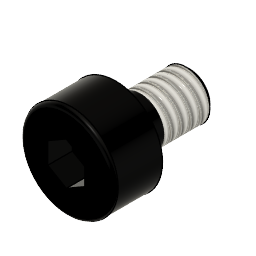
Mesh_Node (Autodesk Fusion 360 archive; units mm, degrees)
design "Hexagon Socket Head Cap Screw ISO 4762 - M2 x 3 Steel 4.6 Black"
description: Hexagon Socket Head Cap Screw ISO 4762 - M2 x 3
part number: ISO 4762 - M2 x 3 Steel 4.6 Black
Autodesk Fusion 360 part; units mm, degrees
sketch "Sketch1" plane through (0, 0, 0) normal (0, 1, 0) x (1, 0, 0)
  line L0 (-1, 0) -> (-1, 3)
  line L1 (-1, 3) -> (0, 3)
  line L2 (0, 3) -> (0, -2)
  line L3 (-1, 0) -> (-1.9, 0)
  line L4 (-1.9, 0) -> (-1.9, -2)
  line L5 (-1.9, -2) -> (0, -2)
  dimension "d9" = 2
  dimension "d106" = 2
  dimension "d107" = 3
  dimension "d116" = 3.8
  constraint perpendicular L0 L1
  constraint collinear origin L1.end L2.end
  constraint perpendicular L0 L3
  constraint coincident origin L3
  constraint vertical L2
  constraint coincident L2 L5.end
  constraint perpendicular L2 L5
  measures "d106" distance of L3 L5
  measures "d107" distance of origin L1
revolve "Revolve1" add sketch "Sketch1" angle 360 about axis through (0, 0, -3) along (0, 0, 1)
ref_plane "WorkPlane1" through (0, 0, 2) normal (0, 0, 1) x (1, 0, 0)
sketch "Sketch6" plane through (0, 0, 2) normal (0, 0, 1) x (1, 0, 0)
  line L0 (-0.75, 0.433) -> (-0.75, -0.433)
  line L1 (-0.75, -0.433) -> (0, -0.866)
  line L2 (0, -0.866) -> (0.75, -0.433)
  line L3 (0.75, -0.433) -> (0.75, 0.433)
  line L4 (0.75, 0.433) -> (0, 0.866)
  line L5 (0, 0.866) -> (-0.75, 0.433)
  dimension "d117" = 1.5
  constraint vertical L0
  measures "d117" distance of L0 L3
extrude "Extrude1" cut sketch "Sketch6" against normal blind 1
extrude "Extrude2" cut 1 faces at (0, -0.2887, 1) along direction (0, 0, -1) blind 1 draft -85
fillet "Fillet4" radius 0.2 1 edges at (-1.7714, 0.6871, 2)
thread "Thread3" "ISO Metric profile 2.0 M2x0.4 M2x0.4 6g" major diameter 1.9335 minor diameter 1.478 pitch 0.4 angle 60 resizes the face on face at (-0.995, 0.0996, -2) from (0, 0, -1) to (0, 0, -3)
sketch "Sketch7" plane through (0, 0, 0) normal (0, 1, 0) x (1, 0, 0)
  line L0 (-1.02, 3) -> (-1.02, 2.8)
  line L1 (-1.02, 2.8) -> (-0.82, 3)
  line L2 (0, 3) -> (0, -2)
  line L3 (-1.02, 3) -> (0, 3)
  dimension "d101" = 45
  dimension "d112" = 0.2
  dimension "d113" = 1.02
  constraint coincident L2.start L3.end
  constraint perpendicular L2 L3
  constraint coincident L1.end L3
  constraint perpendicular L0 L3
  measures "d101" angle of L0 L1
  measures "d112" distance of L0.end L3
  measures "d113" distance of L0 L2.start
revolve "Revolve3" cut sketch "Sketch7" angle 360 about axis through (0, 0, 1.75) along (0, 0, 1)
equation "d9 = adsk_nomdia"
equation "adsk_nomlen = 3.00 mm"
equation "adsk_headh = 2.00 mm"
equation "adsk_headdia = 3.80 mm"
equation "adsk_nomdia = 2.00 mm"
equation "adsk_philwidth = 1.50 mm"
equation "d31 = -adsk_phildepth"
equation "adsk_phildepth = 1.00 mm"
equation "d71 = adsk_headh"
equation "d76 = -adsk_phildepth"
equation "adsk_thrlen = 2.00 mm"
equation "d86 = adsk_nomdia * 0.1"
equation "adsk_startang = 45.00 deg"
equation "d101 = adsk_startang"
equation "adsk_pitch1 = 0.40 mm"
equation "adsk_startlen = 0.20 mm"
equation "d106 = adsk_headh"
equation "d107 = adsk_nomlen"
equation "d112 = adsk_startlen"
equation "d113 = adsk_nomdia * 0.51"
equation "d115 = min(adsk_thrlen; adsk_nomlen - 0.001 mm)"
equation "d116 = adsk_headdia"
equation "d117 = adsk_philwidth"

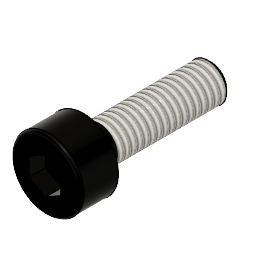
design "Hexagon Socket Head Cap Screw ISO 4762 - M3 x 10 Steel 4.6 Black"
description: Hexagon Socket Head Cap Screw ISO 4762 - M3 x 10
part number: ISO 4762 - M3 x 10 Steel 4.6 Black
Autodesk Fusion 360 part; units mm, degrees
sketch "Sketch1" plane through (0, 0, 0) normal (0, 1, 0) x (1, 0, 0)
  line L0 (-1.5, 0) -> (-1.5, 10)
  line L1 (-1.5, 10) -> (0, 10)
  line L2 (0, 10) -> (0, -3)
  line L3 (-1.5, 0) -> (-2.75, 0)
  line L4 (-2.75, 0) -> (-2.75, -3)
  line L5 (-2.75, -3) -> (0, -3)
  dimension "d9" = 3
  dimension "d106" = 3
  dimension "d107" = 10
  dimension "d116" = 5.5
  constraint perpendicular L0 L1
  constraint collinear origin L1.end L2.end
  constraint perpendicular L0 L3
  constraint coincident origin L3
  constraint vertical L2
  constraint coincident L2 L5.end
  constraint perpendicular L2 L5
  measures "d106" distance of L3 L5
  measures "d107" distance of origin L1
revolve "Revolve1" add sketch "Sketch1" angle 360 about axis through (0, 0, -10) along (0, 0, 1)
ref_plane "WorkPlane1" through (0, 0, 3) normal (0, 0, 1) x (1, 0, 0)
sketch "Sketch6" plane through (0, 0, 3) normal (0, 0, 1) x (1, 0, 0)
  line L0 (-1.25, 0.7217) -> (-1.25, -0.7217)
  line L1 (-1.25, -0.7217) -> (0, -1.4434)
  line L2 (0, -1.4434) -> (1.25, -0.7217)
  line L3 (1.25, -0.7217) -> (1.25, 0.7217)
  line L4 (1.25, 0.7217) -> (0, 1.4434)
  line L5 (0, 1.4434) -> (-1.25, 0.7217)
  dimension "d117" = 2.5
  constraint vertical L0
  measures "d117" distance of L0 L3
extrude "Extrude1" cut sketch "Sketch6" against normal blind 1.3
extrude "Extrude2" cut 1 faces at (0, -0.4811, 1.7) along direction (0, 0, -1) blind 1.3 draft -85
fillet "Fillet4" radius 0.3 1 edges at (-2.5639, 0.9944, 3)
thread "Thread3" "ISO Metric profile 3.0 M3x0.5 M3x0.5 6g" major diameter 2.927 minor diameter 2.3555 pitch 0.5 angle 60 resizes the face on face at (-1.4925, 0.1494, -6.6667) from (0, 0, -1.25) to (0, 0, -10)
sketch "Sketch7" plane through (0, 0, 0) normal (0, 1, 0) x (1, 0, 0)
  line L0 (-1.53, 10) -> (-1.53, 9.7)
  line L1 (-1.53, 9.7) -> (-1.23, 10)
  line L2 (0, 10) -> (0, -3)
  line L3 (-1.53, 10) -> (0, 10)
  dimension "d101" = 45
  dimension "d112" = 0.3
  dimension "d113" = 1.53
  constraint coincident L2.start L3.end
  constraint perpendicular L2 L3
  constraint coincident L1.end L3
  constraint perpendicular L0 L3
  measures "d101" angle of L0 L1
  measures "d112" distance of L0.end L3
  measures "d113" distance of L0 L2.start
revolve "Revolve3" cut sketch "Sketch7" angle 360 about axis through (0, 0, 1.75) along (0, 0, 1)
equation "d9 = adsk_nomdia"
equation "adsk_nomlen = 10.00 mm"
equation "adsk_headh = 3.00 mm"
equation "adsk_headdia = 5.50 mm"
equation "adsk_nomdia = 3.00 mm"
equation "adsk_philwidth = 2.50 mm"
equation "d31 = -adsk_phildepth"
equation "adsk_phildepth = 1.30 mm"
equation "d71 = adsk_headh"
equation "d76 = -adsk_phildepth"
equation "adsk_thrlen = 8.75 mm"
equation "d86 = adsk_nomdia * 0.1"
equation "adsk_startang = 45.00 deg"
equation "d101 = adsk_startang"
equation "adsk_pitch1 = 0.50 mm"
equation "adsk_startlen = 0.30 mm"
equation "d106 = adsk_headh"
equation "d107 = adsk_nomlen"
equation "d112 = adsk_startlen"
equation "d113 = adsk_nomdia * 0.51"
equation "d115 = min(adsk_thrlen; adsk_nomlen - 0.001 mm)"
equation "d116 = adsk_headdia"
equation "d117 = adsk_philwidth"

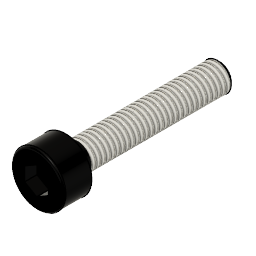
design "Hexagon Socket Head Cap Screw ISO 4762 - M3 x 16 Steel 4.6 Black"
description: Hexagon Socket Head Cap Screw ISO 4762 - M3 x 16
part number: ISO 4762 - M3 x 16 Steel 4.6 Black
Autodesk Fusion 360 part; units mm, degrees
sketch "Sketch1" plane through (0, 0, 0) normal (0, 1, 0) x (1, 0, 0)
  line L0 (-1.5, 0) -> (-1.5, 16)
  line L1 (-1.5, 16) -> (0, 16)
  line L2 (0, 16) -> (0, -3)
  line L3 (-1.5, 0) -> (-2.75, 0)
  line L4 (-2.75, 0) -> (-2.75, -3)
  line L5 (-2.75, -3) -> (0, -3)
  dimension "d9" = 3
  dimension "d106" = 3
  dimension "d107" = 16
  dimension "d116" = 5.5
  constraint perpendicular L0 L1
  constraint collinear origin L1.end L2.end
  constraint perpendicular L0 L3
  constraint coincident origin L3
  constraint vertical L2
  constraint coincident L2 L5.end
  constraint perpendicular L2 L5
  measures "d106" distance of L3 L5
  measures "d107" distance of origin L1
revolve "Revolve1" add sketch "Sketch1" angle 360 about axis through (0, 0, -16) along (0, 0, 1)
ref_plane "WorkPlane1" through (0, 0, 3) normal (0, 0, 1) x (1, 0, 0)
sketch "Sketch6" plane through (0, 0, 3) normal (0, 0, 1) x (1, 0, 0)
  line L0 (-1.25, 0.7217) -> (-1.25, -0.7217)
  line L1 (-1.25, -0.7217) -> (0, -1.4434)
  line L2 (0, -1.4434) -> (1.25, -0.7217)
  line L3 (1.25, -0.7217) -> (1.25, 0.7217)
  line L4 (1.25, 0.7217) -> (0, 1.4434)
  line L5 (0, 1.4434) -> (-1.25, 0.7217)
  dimension "d117" = 2.5
  constraint vertical L0
  measures "d117" distance of L0 L3
extrude "Extrude1" cut sketch "Sketch6" against normal blind 1.3
extrude "Extrude2" cut 1 faces at (0, -0.4811, 1.7) along direction (0, 0, -1) blind 1.3 draft -85
fillet "Fillet4" radius 0.3 1 edges at (-2.5639, 0.9944, 3)
thread "Thread3" "ISO Metric profile 3.0 M3x0.5 M3x0.5 6g" major diameter 2.927 minor diameter 2.3555 pitch 0.5 angle 60 resizes the face on face at (-1.4925, 0.1494, -10.6667) from (0, 0, -1.25) to (0, 0, -16)
sketch "Sketch7" plane through (0, 0, 0) normal (0, 1, 0) x (1, 0, 0)
  line L0 (-1.53, 16) -> (-1.53, 15.7)
  line L1 (-1.53, 15.7) -> (-1.23, 16)
  line L2 (0, 16) -> (0, -3)
  line L3 (-1.53, 16) -> (0, 16)
  dimension "d101" = 45
  dimension "d112" = 0.3
  dimension "d113" = 1.53
  constraint coincident L2.start L3.end
  constraint perpendicular L2 L3
  constraint coincident L1.end L3
  constraint perpendicular L0 L3
  measures "d101" angle of L0 L1
  measures "d112" distance of L0.end L3
  measures "d113" distance of L0 L2.start
revolve "Revolve3" cut sketch "Sketch7" angle 360 about axis through (0, 0, 1.75) along (0, 0, 1)
equation "d9 = adsk_nomdia"
equation "adsk_nomlen = 16.00 mm"
equation "adsk_headh = 3.00 mm"
equation "adsk_headdia = 5.50 mm"
equation "adsk_nomdia = 3.00 mm"
equation "adsk_philwidth = 2.50 mm"
equation "d31 = -adsk_phildepth"
equation "adsk_phildepth = 1.30 mm"
equation "d71 = adsk_headh"
equation "d76 = -adsk_phildepth"
equation "adsk_thrlen = 14.75 mm"
equation "d86 = adsk_nomdia * 0.1"
equation "adsk_startang = 45.00 deg"
equation "d101 = adsk_startang"
equation "adsk_pitch1 = 0.50 mm"
equation "adsk_startlen = 0.30 mm"
equation "d106 = adsk_headh"
equation "d107 = adsk_nomlen"
equation "d112 = adsk_startlen"
equation "d113 = adsk_nomdia * 0.51"
equation "d115 = min(adsk_thrlen; adsk_nomlen - 0.001 mm)"
equation "d116 = adsk_headdia"
equation "d117 = adsk_philwidth"

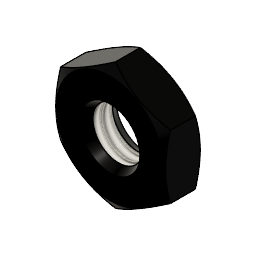
design "Hexagon Thin Nut ISO 4035 - M3 Steel 6 Black"
description: Hexagon Thin Nut ISO 4035 - M3
part number: ISO 4035 - M3 Steel 6 Black
Autodesk Fusion 360 part; units mm, degrees
sketch "Sketch1" plane through (0, 0, 0) normal (0, 1, 0) x (1, 0, 0)
  line L0 (0, 0) -> (0, -1.8)
  line L1 (-1.5, 0) -> (-2.695, 0)
  line L2 (-2.695, 0) -> (-3.1763, -0.2778)
  line L3 (-3.1763, -0.2778) -> (-3.1763, -1.5222)
  line L4 (-3.1763, -1.5222) -> (-2.695, -1.8)
  line L5 (-2.695, -1.8) -> (-1.5, -1.8)
  line L6 (-1.5, -1.8) -> (-1.5, 0)
  dimension "d121" = 3
  dimension "d122" = 30
  dimension "d123" = 30
  dimension "d128" = 6.3525
  dimension "d172" = 5.39
  dimension "d179" = 1.8
  constraint vertical L0
  constraint coincident L0 L0.end
  constraint coincident origin L0
  constraint horizontal L1
  constraint coincident L0.start L1
  constraint coincident L0.start origin
  constraint coincident L0.end L5
  constraint vertical L1.end L4.end
  measures "d122" angle of L1 L2
  measures "d123" angle of L4 L5
  measures "d179" distance of L1 L5
revolve "Revolve1" add sketch "Sketch1" angle 360 about axis through (0, 0, 0) along (0, 0, 1)
sketch "Sketch8" plane through (0, 0, 1.8) normal (0, 0, 1) x (1, 0, 0)
  line L0 (-2.75, -1.5894) -> (-2.75, 1.5894)
  circle A0 centre (0, 0) radius 1.5
  circle A1 centre (0, 0) radius 3.1763
  dimension "d114" = 2.75
  constraint coincident L0.end A1
  constraint coincident L0.start A1
  constraint vertical L0
  measures "d114" distance of A0.centre L0
extrude "Extrude5" cut sketch "Sketch8" against normal blind 1.8 contours L0 A1 picked at (-2.8188, -0.3871)
pattern_circular "C-Pattern2" count 6 over 360 about axis through (0, 0, 1.75) along (0, 0, 1) of "Extrude5"
thread "Thread3" "ISO Metric profile 3.0 M3x0.5 M3x0.5 6H" major diameter 3.086 minor diameter 2.529 pitch 0.5 angle 60 resizes the face on face at (-1.4981, 0.0748, 1.2)
sketch "Sketch12" plane through (0, 0, 0) normal (0, 1, 0) x (1, 0, 0)
  line L0 (-1.5, 0) -> (0, 0)
  line L1 (-0.9804, -0.9) -> (-1.5, 0)
  line L2 (-1.5, -1.8) -> (0, -1.8)
  line L3 (-0.9804, -0.9) -> (-1.5, -1.8)
  line L4 (0, 0) -> (0, -1.8)
  dimension "d169" = 60
  dimension "d177" = 1.5
  dimension "d178" = 60
  constraint horizontal L0
  constraint coincident L1.start L3.start
  constraint vertical L0.start L2.start
  constraint coincident L2.end L4.end
  constraint coincident L0.end L4.start
  constraint perpendicular L2 L4
  measures "d169" angle of L2 L3
  measures "d177" distance of L0.start L4
  measures "d178" angle of L0 L1
revolve "Revolve3" cut sketch "Sketch12" angle 360 about axis through (0, 0, 1.75) along (0, 0, 1)
equation "adsk_nheig = 1.80 mm"
equation "adsk_maxdia = 6.3525 mm"
equation "adsk_nomdia = 3.00 mm"
equation "d89 = -adsk_nheig"
equation "adsk_waflat = 5.50 mm"
equation "d114 = adsk_waflat / 2"
equation "adsk_chamang1 = 30.00 deg"
equation "adsk_chamang2 = 30.00 deg"
equation "d121 = adsk_nomdia"
equation "d122 = adsk_chamang1"
equation "d123 = adsk_chamang2"
equation "d128 = adsk_maxdia"
equation "d163 = adsk_nheig"
equation "adsk_beardia = 5.39 mm"
equation "d172 = adsk_beardia"
equation "d177 = adsk_nomdia * 0.5"
equation "d179 = adsk_nheig"

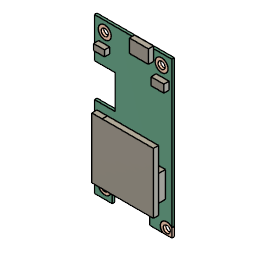
design "RAK19007"
Autodesk Fusion 360 part; units mm, degrees
sketch "Sketch1" plane through (0, 0, 0) normal (0, 0, 1) x (1, 0, 0)
  line L0 (-15, 30) -> (15, 30)
  line L1 (15, 30) -> (15, -30)
  line L2 (15, -30) -> (-15, -30)
  line L3 (-15, -30) -> (-15, 30)
  line L4 (0, 0) -> (0, 30) construction
  line L5 (0, 0) -> (-15, 0) construction
  circle A0 centre (-11, 26) radius 1.35
  circle A1 centre (-11, 26) radius 2.5
  line L6 (-11, 26) -> (-11, 30) construction
  line L7 (-11, 26) -> (-15, 26) construction
  circle A2 centre (11, 26) radius 1.35
  circle A3 centre (11, 26) radius 2.5
  line L8 (0.5492, 25.7284) -> (7.9022, 25.7284)
  line L9 (7.9022, 25.7284) -> (7.9022, 30.9089)
  line L10 (7.9022, 30.9089) -> (0.5492, 30.9089)
  line L11 (0.5492, 30.9089) -> (0.5492, 25.7284)
  line L12 (8.9383, 22.0853) -> (13.8849, 22.0853)
  line L13 (13.8849, 22.0853) -> (13.8849, 19.0773)
  line L14 (13.8849, 19.0773) -> (8.9383, 19.0773)
  line L15 (8.9383, 19.0773) -> (8.9383, 22.0853)
  line L16 (-13.3546, 22.0853) -> (-9.0765, 22.0853)
  line L17 (-9.0765, 22.0853) -> (-9.0765, 19.7457)
  line L18 (-9.0765, 19.7457) -> (-13.3546, 19.7457)
  line L19 (-13.3546, 19.7457) -> (-13.3546, 22.0853)
  line L20 (-15, 14.5) -> (-7, 14.5)
  line L21 (-7, 14.5) -> (-7, 1.5)
  line L22 (-7, 1.5) -> (-15, 1.5)
  circle A4 centre (-11, -26) radius 2.5
  circle A5 centre (-11, -26) radius 1.35
  circle A6 centre (13, -28) radius 1.35
  circle A7 centre (13, -28) radius 2.5
  line L23 (-11, -26) -> (-11, -30) construction
  line L24 (-11, -26) -> (-15, -26) construction
  line L25 (11, 26) -> (15, 26) construction
  line L26 (13, -28) -> (15, -28) construction
  line L27 (13, -28) -> (13, -30) construction
  line L28 (-8.1, -30) -> (-8.1, -22)
  line L29 (-8.1, -22) -> (6.4, -22)
  line L30 (6.4, -22) -> (6.4, -30)
  line L31 (10, -8.2) -> (12.5, -8.2)
  line L32 (12.5, -8.2) -> (12.5, -18.2)
  line L33 (12.5, -18.2) -> (10, -18.2)
  line L34 (10, -18.2) -> (10, -8.2)
  line L35 (10, -13.2) -> (-15, -13.2) construction
  line L36 (-11.0289, 1.517) -> (12.837, 1.517)
  line L37 (12.837, 1.517) -> (12.837, -21.9402)
  line L38 (12.837, -21.9402) -> (-11.0289, -21.9402)
  line L39 (-11.0289, -21.9402) -> (-11.0289, 1.517)
  dimension "d1" = 30
  dimension "d2" = 60
  dimension "d3" = 5
  dimension "d4" = 2.7
  dimension "d5" = 4
  dimension "d6" = 5
  dimension "d7" = 2.7
  dimension "d8" = 22
  dimension "d9" = 13
  dimension "d10" = 15.5
  dimension "d11" = 8
  dimension "d13" = 52
  dimension "d14" = 2
  dimension "d15" = 2
  dimension "d16" = 8
  dimension "d17" = 14.5
  dimension "d18" = 6.9
  dimension "d27" = 2.5
  dimension "d28" = 10
  dimension "d29" = 39.2
  dimension "d30" = 2.5
  constraint horizontal L0
  constraint vertical L1
  constraint horizontal L2
  constraint vertical L3
  constraint coincident L4.start L5.start
  constraint midpoint L0 L4.end
  constraint midpoint L3 L5.end
  constraint vertical L4
  constraint horizontal L5
  constraint concentric A0 A1
  constraint coincident A0.centre A1.centre
  constraint coincident L0 L6.end
  constraint perpendicular L0 L6
  constraint coincident L3 L7.end
  constraint perpendicular L3 L7
  constraint equal L6 L7
  constraint concentric A2 A3
  constraint horizontal L8
  constraint vertical L9
  constraint horizontal L10
  constraint vertical L11
  constraint horizontal L12
  constraint vertical L13
  constraint horizontal L14
  constraint vertical L15
  constraint horizontal L16
  constraint vertical L17
  constraint horizontal L18
  constraint vertical L19
  constraint coincident L3 L20.start
  constraint perpendicular L3 L20
  constraint perpendicular L20 L21
  constraint coincident L3 L22.end
  constraint perpendicular L3 L22
  constraint concentric A4 A5
  constraint equal A0 A5
  constraint equal A1 A4
  constraint concentric A6 A7
  constraint coincident A4.centre A5.centre
  constraint coincident L2 L23.end
  constraint perpendicular L2 L23
  constraint coincident L3 L24.end
  constraint perpendicular L3 L24
  constraint collinear L6 L23
  constraint coincident A2.centre A3.centre
  constraint coincident L1 L25.end
  constraint perpendicular L1 L25
  constraint collinear L7 L25
  constraint coincident A6.centre A7.centre
  constraint coincident L1 L26.end
  constraint perpendicular L1 L26
  constraint coincident L2 L27.end
  constraint perpendicular L2 L27
  constraint coincident L2 L28.start
  constraint perpendicular L2 L28
  constraint perpendicular L28 L29
  constraint coincident L2 L30.end
  constraint perpendicular L2 L30
  constraint equal A5 A6
  constraint equal A4 A7
  constraint horizontal L31
  constraint vertical L32
  constraint horizontal L33
  constraint vertical L34
  constraint midpoint L34 L35.start
  constraint coincident L3 L35.end
  constraint perpendicular L3 L35
  constraint horizontal L36
  constraint vertical L37
  constraint horizontal L38
  constraint vertical L39
  measures "d1" distance of L0.start L0.end
  measures "d2" distance of L0.start L2.end
  measures "d3" diameter of A1
  measures "d4" diameter of A0
  measures "d5" distance of A0.centre L7.end
  measures "d6" diameter of A3
  measures "d7" diameter of A2
  measures "d8" distance of A0.centre A2.centre
  measures "d9" distance of L20 L22
  measures "d10" distance of L0 L20
  measures "d11" distance of L20.start L20.end
  measures "d13" distance of L7 L24
  measures "d14" distance of L2 L26
  measures "d15" distance of L1 L27
  measures "d16" distance of L2 L29
  measures "d17" distance of L28 L30
  measures "d18" distance of L3 L28
  measures "d27" distance of L31.start L31.end
  measures "d28" distance of L31.start L33.end
  measures "d29" distance of L7 L35
  measures "d30" distance of L1 L32
extrude "Extrude1" add sketch "Sketch1" along normal blind 1 contours L0 L1 L2 L3 L8 L9 L11 L20 L21 L22 A7 L28 L29 L30 L36 L37 L38 L39 | L0 L8 L9 L11 | L21 L22 L36 L37 L38 L39 | L12 L13 L14 L15 | L16 L17 L18 L19 | L31 L32 L33 L34 makes body 1
extrude "Extrude2" add sketch "Sketch1" along normal blind 1 separate body contours L1 L2 A7 | L1 L2 A7 | A1 | A3 | A4 makes body 2 at (13.4969, 25.8754, 0.6667) makes body 3 at (-8.5031, -26.1246, 0.6667) makes body 4 at (-8.5031, 25.8754, 0.6667) makes body 5 at (13.2003, -29.7821, 0)
extrude "Extrude3" add sketch "Sketch1" along normal blind 2 from surface at 1 separate body contours L0 L9 L10 L11 | L0 L8 L9 L11 | L12 L13 L14 L15 | L16 L17 L18 L19 makes body 6 at (3.0002, 27.4553, 1) makes body 7 at (12.2361, 20.08, 1) makes body 8 at (-11.9286, 21.3055, 1)
extrude "Extrude4" add sketch "Sketch1" along normal blind 3 from surface at 1 separate body contours L31 L32 L33 L34 makes body 9
extrude "Extrude5" add sketch "Sketch1" along normal blind 2 from surface at 4 separate body contours L21 L22 L36 L37 L38 L39 | L31 L32 L33 L34 makes body 10
equation "d28 = ( 2.5 * 4 ) * 1 mm"

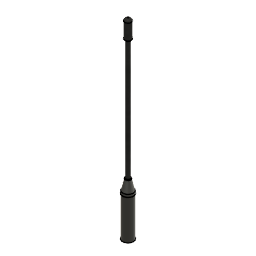
design "915MHz Antenna - Muzi Works"
Autodesk Fusion 360 part; units mm, degrees
sketch "Sketch1" plane through (0, 0, 0) normal (0, 1, 0) x (1, 0, 0)
  circle A0 centre (0, 0) radius 5
  circle A1 centre (0, 0) radius 1.85
  circle A2 centre (0, 0) radius 3
  dimension "d1" = 10
  dimension "d2" = 3.7
  dimension "d3" = 6
  constraint coincident A0.centre A1.centre
  measures "d1" diameter of A0
  measures "d2" diameter of A1
  measures "d3" diameter of A2
extrude "Extrude1" add sketch "Sketch1" along normal blind 48.5 contours A0 | A1 | A2 makes body 1
extrude "Extrude2" add sketch "Sketch1" along normal blind 110 from surface at 48.5 separate body contours A1 makes body 2
extrude "Extrude3" add sketch "Sketch1" along normal blind 18 from surface at 158.5 separate body contours A1 | A2 makes body 3
chamfer "Chamfer1" distance 2.5 distance2 11 1 edges at (-4.6616, 48.5, 1.8081) measured on face at (-1.0946, 48.5, 1.5459) on bodies 1
fillet "Fillet1" radius 0.5 1 edges at (-2.3308, 48.5, -0.904) on bodies 1 3
fillet "Fillet1" radius 10 1 edges at (-4.6616, 37.5, 1.8081) on bodies 1 3
fillet "Fillet1" radius 2.5 1 edges at (-2.797, 176.5, 1.0848) on bodies 1 3
fillet "Fillet1" radius 1.25 1 edges at (-2.797, 158.5, -1.0848) on bodies 1 3
named bodies: "Base", "Antenna", "Rubber cap"
